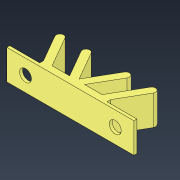
# Autodesk Inventor part: Dribblerdaempfer V2
Saved by Autodesk Inventor 2022.1 (Build 261234020, 234B)
## iProperties
Part Number: Dribblerdaempfer V2
Material: Gummi, Silikon
Document SubType Name: Modeling
Designer: rYan
Mass: 1.4873 g
Surface Area: 21.3602 cm^2
Volume: 1.18984 cm^3
Density: 1.25 g/cm^3
Appearance: Gummi - Schwarz(1)
Author: rYan
Autodesk Inventor part; units mm, degrees
ref_plane "YZ Plane" through (0, 0, 0) normal (1, 0, 0) x (0, 1, 0)
ref_plane "XZ Plane" through (0, 0, 0) normal (0, 1, 0) x (-1, 0, 0)
ref_plane "XY Plane" through (0, 0, 0) normal (0, 0, 1) x (1, 0, 0)
sketch "Skizze1" plane through (0, 0, 0) normal (0, 0, 1) x (1, 0, 0)
  line L0 (-17, 0) -> (17, 0)
  line L1 (0, 2.16) -> (0, -0.36) projected
  line L2 (-17, 0) -> (-17, 0.8)
  line L3 (17, 0.8) -> (17, 0)
  line L4 (-17, 0.8) -> (-9, 0.8)
  line L5 (-9, 0.8) -> (-9, 1.8)
  line L6 (-9, 1.8) -> (9, 1.8)
  line L7 (9, 1.8) -> (9, 0.8)
  line L8 (9, 0.8) -> (17, 0.8)
  point P0 (0, 0)
  dimension "d2" = 0.8
  dimension "d3" = 34
  dimension "d28" = 1
  dimension "d29" = 18
  constraints: 16 end point, 5 perpendicular, 2 vertical, 1 horizontal, 1 midpoint, 3 other
  measures "d2" distance of L2.end L0.start
  measures "d3" distance of L0.start L0.end
  measures "d28" distance of L4.end L5.end
  measures "d29" distance of L5.end L6.end
extrude "Extrusion1" add sketch "Skizze1" along normal blind 8
sketch "Skizze2" plane through (0, 0, 0) normal (0, 0, 1) x (1, 0, 0)
  line L0 (-17, 0) -> (17, 0) construction
  line L1 (17, 0) -> (17, 0.8) construction
  line L2 (-9, 0.8) -> (-17, 0.8) construction
  line L3 (-17, 0.8) -> (-17, 0) construction
  line L4 (-9, 1.8) -> (-13.1569, 9)
  line L5 (-6.6906, 1.8) -> (-9, 1.8)
  line L6 (-6.6906, 1.8) -> (-11.4249, 10)
  arc A0 (-11.4249, 10) -> (-13.1569, 9) centre (-12.2909, 9.5) ccw
  line L7 (-17, 0.8) -> (-17, 0.8) construction
  line L8 (-17, 0.8) -> (-17, 10.5) construction
  line L9 (-17, 10.5) -> (17, 10.5) construction
  line L10 (17, 10.5) -> (17, 0.8) construction
  line L11 (17, 0.8) -> (-9, 0.8) construction
  line L12 (0, 13.8837) -> (0, -2.3139) construction
  arc A1 (-10.865, 10.5) -> (-17, 0.8) centre (-7.8453, 1.8) ccw construction
  line L13 (17, 0.8) -> (9, 0.8) projected
  line L14 (9, 0.8) -> (9, 1.8) projected
  line L15 (9, 1.8) -> (-9, 1.8) construction
  line L16 (-9, 1.8) -> (-9, 0.8) projected
  point P0 (0, 0)
  dimension "d10" = 2
  dimension "d11" = 60
  dimension "d12" = 34
  dimension "d14" = 10.5
  constraints: 16 end point, 4 perpendicular, 4 point on circle, 3 point on line, 3 tangent, 2 centre point, 2 horizontal, 1 midpoint, 1 parallel, 1 other
  measures "d10" distance between parallel lines of L4 L6
  measures "d11" angle of L2 L4
  measures "d12" distance of L8.end L9.end
  measures "d14" distance between parallel lines of L0 L9
extrude "Extrusion2" add sketch "Skizze2" along normal blind 8
pattern_linear "Rechteckige Anordnung1" count 2 spacing 7 along (1, 0, 0) of "Extrusion2"
mirror "Spiegeln1" about plane through (0, 0, 0) normal (1, 0, 0) of "Extrusion2", "Rechteckige Anordnung1"
sketch "Skizze3" plane through (-17, 0, 0) normal (0, -1, 0) x (1, 0, 0)
  line L0 (17, 9.6) -> (17, -1.6) projected
  line L1 (0, 0) -> (34, 0) projected
  line L2 (34, 0) -> (34, 8) projected
  line L3 (0, 8) -> (34, 8) projected
  line L4 (0, 0) -> (0, 8) projected
  line L5 (0, 0) -> (0, 8) construction
  line L6 (0, 4) -> (34, 4) construction
  point P0 (17, 0)
  point P1 (5, 4)
  point P2 (29, 4)
  dimension "d20" = 24
  constraints: 2 end point, 2 midpoint, 1 point on line, 1 symmetric about line
  measures "d20" distance of point (29, 4) point (5, 4)
hole "Bohrung1" at (-12, 0, 4) at (12, 0, 4) direction (0, 1, 0) diameter 3.2 depth 2 tip angle 118
